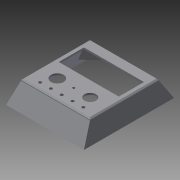
# Autodesk Inventor part: gora_obodowy_plaska
Saved by Autodesk Inventor 2015 SP1 (Build 190203100, 203)
## iProperties
Created: 2015-05-15
Part Number: gora_obodowy_plaska
Material: Ogólny
Document SubType Name: Modeling
Designer: Kuba
Density: 1 g/cm^3
Appearance: Domyślna
Author: Kuba
Autodesk Inventor part; units mm, degrees
ref_plane "YZ Plane" through (0, 0, 0) normal (1, 0, 0) x (0, 1, 0)
ref_plane "XZ Plane" through (0, 0, 0) normal (0, 1, 0) x (-1, 0, 0)
ref_plane "XY Plane" through (0, 0, 0) normal (0, 0, 1) x (1, 0, 0)
sketch "Szkic1" plane through (0, 0, 0) normal (0, 0, 1) x (1, 0, 0)
  line L0 (-55, -55) -> (55, -55)
  line L1 (55, -55) -> (55, 55)
  line L2 (55, 55) -> (-55, 55)
  line L3 (-55, 55) -> (-55, -55)
  line L4 (-55, -55) -> (55, 55) construction
  line L5 (-55, 55) -> (-55, 40) construction
  line L6 (-55, 40) -> (-50, 40)
  line L7 (-50, 40) -> (50, 40)
  line L8 (50, 40) -> (50, -2)
  line L9 (50, -2) -> (-50, -2)
  line L10 (-50, -2) -> (-50, 40)
  line L11 (0, -2) -> (0, -27) construction
  circle A0 centre (0, -27) radius 2
  line L12 (0, -27) -> (27.5, -27) construction
  line L13 (27.5, -27) -> (-27.5, -27) construction
  circle A1 centre (-27.5, -27) radius 10.5
  circle A2 centre (27.5, -27) radius 9.5
  line L14 (0, -27) -> (0, -47) construction
  line L15 (0, -47) -> (0, -57) construction
  line L16 (0, -47) -> (-18, -47) construction
  line L17 (-18, -47) -> (-36, -47) construction
  line L18 (0, -47) -> (18, -47) construction
  line L19 (18, -47) -> (36, -47) construction
  circle A3 centre (-36, -47) radius 2.5
  circle A4 centre (-18, -47) radius 2.5
  circle A5 centre (0, -47) radius 2.5
  circle A6 centre (18, -47) radius 2.5
  circle A7 centre (36, -47) radius 2.5
  line L20 (-57.5, -57.5) -> (57.5, -57.5)
  line L21 (57.5, -57.5) -> (57.5, 57.5)
  line L22 (57.5, 57.5) -> (-57.5, 57.5)
  line L23 (-57.5, 57.5) -> (-57.5, -57.5)
  line L24 (-57.5, -57.5) -> (57.5, 57.5) construction
  line L25 (57.5, -57.5) -> (-57.5, 57.5) construction
  point P0 (0, 0)
  point P1 (-55, -37)
  point P2 (55, -37)
  dimension "d0" = 110
  dimension "d1" = 110
  dimension "d2" = 15
  dimension "d3" = 100
  dimension "d4" = 42
  dimension "d5" = 25
  dimension "d6" = 4
  dimension "d7" = 27.5
  dimension "d8" = 55
  dimension "d10" = 19
  dimension "d11" = 20
  dimension "d12" = 10
  dimension "d13" = 18
  dimension "d14" = 18
  dimension "d15" = 18
  dimension "d16" = 18
  dimension "d17" = 5
  dimension "d18" = 5
  dimension "d19" = 5
  dimension "d20" = 5
  dimension "d21" = 5
  dimension "d51" = 115
  dimension "d52" = 115
  constraints: 52 end point, 8 centre point, 8 coincident, 7 parallel, 6 horizontal, 6 point on line, 5 perpendicular, 4 midpoint, 1 vertical
  measures "d0" distance of L2.end L1.end
  measures "d1" distance of L1.end L0.end
  measures "d2" distance of L2.end L5.end
  measures "d3" distance of L8.end L9.end
  measures "d4" distance of L7.end L8.end
  measures "d5" distance of L11.start L11.end
  measures "d6" diameter of A0
  measures "d7" distance of L12.start L12.end
  measures "d8" distance of L12.end L13.end
  measures "d10" diameter of A2
  measures "d11" distance of L12.start L14.end
  measures "d12" distance of L14.end L15.end
  measures "d13" distance of L14.end L16.end
  measures "d14" distance of L16.end L17.end
  measures "d15" distance of L14.end L18.end
  measures "d16" distance of L18.end L19.end
  measures "d17" diameter of A3
  measures "d18" diameter of A4
  measures "d19" diameter of A5
  measures "d20" diameter of A6
  measures "d21" diameter of A7
  measures "d51" distance of L22.end L21.end
  measures "d52" distance of L21.end L20.end
extrude "Wyciągnięcie proste1" add sketch "Szkic1" along normal blind 3 contours L3 L2 L1 L0 | L23 L22 L21 L20
ref_plane "Płaszczyzna konstrukcyjna1" through (0, 0, -30) normal (0, 0, -1) x (-1, 0, 0)
ref_plane "Płaszczyzna konstrukcyjna2" through (0, 0, -20) normal (0, 0, -1) x (-1, 0, 0)
ref_plane "Płaszczyzna konstrukcyjna3" through (0, 0, 0) normal (0, 0, -1) x (-1, 0, 0)
ref_plane "Płaszczyzna konstrukcyjna4" through (75, -75, -30) normal (0, 0, -1) x (-1, 0, 0)
chamfer "Faza1" distance 2 angle 45 4 edges at (0, 57.5, 3) (-57.5, 0, 3) (57.5, 0, 3) (0, -57.5, 3)
sketch "Szkic9" plane through (0, 0, 0) normal (0, 0, -1) x (-1, 0, 0)
  line L0 (-57.5, -57.5) -> (57.5, -57.5)
  line L1 (57.5, -57.5) -> (57.5, 57.5)
  line L2 (57.5, 57.5) -> (-57.5, 57.5)
  line L3 (-57.5, 57.5) -> (-57.5, -57.5)
  line L4 (-57.5, -57.5) -> (57.5, 57.5) construction
  line L5 (57.5, -57.5) -> (-57.5, 57.5) construction
  point P0 (0, 0)
  constraints: 12 end point, 2 midpoint, 2 parallel, 1 horizontal, 1 perpendicular
sketch "Szkic10" plane through (0, 0, 0) normal (0, 0, -1) x (-1, 0, 0)
  line L0 (-55, -55) -> (55, -55)
  line L1 (55, -55) -> (55, 55)
  line L2 (55, 55) -> (-55, 55)
  line L3 (-55, 55) -> (-55, -55)
  line L4 (-55, -55) -> (55, 55) construction
  line L5 (55, -55) -> (-55, 55) construction
  point P0 (0, 0)
  dimension "d67" = 110
  dimension "d68" = 110
  constraints: 12 end point, 2 midpoint, 2 parallel, 1 horizontal, 1 perpendicular
  measures "d67" distance of L2.end L1.end
  measures "d68" distance of L1.end L0.end
ref_plane "Płaszczyzna konstrukcyjna5" through (45.0845, 55, -30) normal (0, 0, -1) x (-1, 0, 0)
sketch "Szkic14" plane through (45.0845, 55, -30) normal (0, 0, -1) x (-1, 0, 0)
  line L0 (-19.9155, -130) -> (110.0845, -130)
  line L1 (110.0845, -130) -> (110.0845, 20)
  line L2 (110.0845, 20) -> (-19.9155, 20)
  line L3 (-19.9155, 20) -> (-19.9155, -130)
  line L4 (-19.9155, -130) -> (110.0845, 20) construction
  line L5 (110.0845, -130) -> (-19.9155, 20) construction
  point P0 (45.0845, -55)
  dimension "d93" = 130
  dimension "d94" = 150
  constraints: 12 end point, 2 midpoint, 2 parallel, 1 horizontal, 1 perpendicular
  measures "d93" distance of L2.end L1.end
  measures "d94" distance of L1.end L0.end
sketch "Szkic15" plane through (45.0845, 55, -30) normal (0, 0, -1) x (-1, 0, 0)
  line L0 (107.5845, -127.5) -> (-17.4155, -127.5)
  line L1 (-17.4155, -127.5) -> (-17.4155, 17.5)
  line L2 (-17.4155, 17.5) -> (107.5845, 17.5)
  line L3 (107.5845, 17.5) -> (107.5845, -127.5)
  line L4 (107.5845, -127.5) -> (-17.4155, 17.5) construction
  line L5 (-17.4155, -127.5) -> (107.5845, 17.5) construction
  point P0 (45.0845, -55)
  dimension "d95" = 125
  dimension "d96" = 145
  constraints: 12 end point, 2 midpoint, 2 parallel, 1 horizontal, 1 perpendicular
  measures "d95" distance of L1.end L2.end
  measures "d96" distance of L0.end L1.end
loft "Wyciągnięcie złożone5" add profiles "Szkic9", "Szkic14"
loft "Wyciągnięcie złożone6" cut profiles "Szkic15", "Szkic10"
sketch "Szkic8" plane through (0, 0, -20) normal (0, 0, -1) x (-1, 0, 0)
  line L0 (-52.5, -52.5) -> (52.5, 52.5) construction
  line L1 (-55, 55) -> (-62.5, 72.5) projected
  line L2 (52.5, 52.5) -> (52.5, 47.5)
  line L3 (52.5, 47.5) -> (38.6222, 60.8006)
  line L4 (57.5113, 42.6971) -> (52.5, 47.5)
  line L5 (-52.5, 52.5) -> (-47.5006, 52.5806)
  line L6 (-47.5006, 52.5806) -> (-33.6043, 66.9631)
  line L7 (-47.5006, 52.5806) -> (-60.6627, 38.958)
  line L8 (-60.6627, 38.958) -> (-60.1271, 66.9631)
  line L9 (-60.1271, 66.9631) -> (-33.6043, 66.9631)
  line L10 (-52.5, -52.5) -> (-42.5, -52.5)
  line L11 (-42.5, -52.5) -> (-60.3532, -35.2504)
  line L12 (45.4959, -47.1074) -> (40.6649, -52.1074)
  line L13 (45.4959, -47.1074) -> (60.2173, -31.8709)
  line L14 (-60.3532, -35.2504) -> (-60.3532, -67.4907)
  line L15 (-55, -55) -> (-62.5, -72.5) projected
  line L16 (-42.5, -52.5) -> (-34.5509, -60.4491)
  line L17 (-42.5, -52.5) -> (-31.2582, -52.5) construction
  line L18 (-60.3532, -67.4907) -> (-27.5093, -67.4907)
  line L19 (-27.5093, -67.4907) -> (-35.5667, -59.4333)
  line L20 (57.5113, 42.6971) -> (38.6222, 60.8006)
  line L21 (38.6222, 60.8006) -> (32.1923, 66.9631)
  line L22 (32.1923, 66.9631) -> (60.2173, 66.9631)
  line L23 (60.2173, 66.9631) -> (60.4778, 39.854)
  line L24 (60.4778, 39.854) -> (57.5113, 42.6971)
  line L25 (40.6649, -52.1074) -> (27.9311, -65.2867)
  line L26 (27.9311, -65.2867) -> (61.4401, -66.3113)
  line L27 (60.2173, -31.8709) -> (61.4401, -66.3113)
  point P0 (0, 0)
  dimension "d83" = 5
  dimension "d84" = 5
  dimension "d85" = 10
  dimension "d87" = 45
  constraints: 52 end point, 8 point on line, 3 collinear, 3 horizontal, 2 perpendicular, 1 equal length, 1 midpoint, 1 vertical
  measures "d83" distance of L0.end L2.end
  measures "d84" distance of L5.start L5.end
  measures "d85" distance of L0.start L10.end
  measures "d87" angle of L16 L17
extrude "Wyciągnięcie proste3" add sketch "Szkic8" against normal up to next
